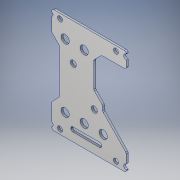
# Autodesk Inventor part: End Plate - 18S
Saved by Autodesk Inventor 2017 (Build 210142000, 142)
## iProperties
Created: 2021-03-03
Part Number: End Plate - 18S
Material: Aluminum 6061
Document SubType Name: Modeling
Designer: Win240
Density: 2.7 g/cm^3
Appearance: Aluminum - Flat
Mass: 164.512 g
Surface Area: 306.178 cm^2
Volume: 60.9303 cm^3
Author: Win240
Autodesk Inventor part; units mm, degrees
ref_plane "YZ Plane" through (0, 0, 0) normal (1, 0, 0) x (0, 1, 0)
ref_plane "XZ Plane" through (0, 0, 0) normal (0, 1, 0) x (-1, 0, 0)
ref_plane "XY Plane" through (0, 0, 0) normal (0, 0, 1) x (1, 0, 0)
sketch "Sketch1" plane through (0, 0, 0) normal (0, 0, 1) x (1, 0, 0)
  line L0 (0, 0) -> (119, 0)
  line L1 (119, 0) -> (119, -24.5)
  line L2 (119, -165) -> (0, -165)
  line L3 (0, -165) -> (0, 0)
  arc A0 (0, -11.373) -> (0, -3.627) centre (-1, -7.5) ccw
  arc A1 (119, -3.627) -> (119, -11.373) centre (120, -7.5) ccw
  arc A2 (119, -153.627) -> (119, -161.373) centre (120, -157.5) ccw
  arc A3 (0, -161.373) -> (0, -153.627) centre (-1, -157.5) ccw
  line L4 (-1, -7.5) -> (120, -7.5) construction
  line L5 (120, -7.5) -> (120, -157.5) construction
  line L6 (120, -157.5) -> (-1, -157.5) construction
  line L7 (-1, -157.5) -> (-1, -7.5) construction
  line L8 (-1, -7.5) -> (0, -3.627) construction
  line L9 (120, -7.5) -> (119, -3.627) construction
  line L10 (59.5, -7.5) -> (59.5, 0) construction
  line L11 (59.5, -157.5) -> (59.5, -165) construction
  circle A4 centre (22, -31) radius 6.5
  circle A5 centre (52, -31) radius 6.5
  arc A6 (82, -24.5) -> (78.25, -36.3092) centre (82, -31) ccw
  circle A7 centre (82, -131) radius 6.5
  circle A8 centre (52, -131) radius 6.5
  circle A9 centre (22, -131) radius 6.5
  line L12 (22, -31) -> (52, -31) construction
  line L13 (52, -31) -> (82, -31) construction
  line L14 (82, -31) -> (82, -131) construction
  line L15 (82, -131) -> (52, -131) construction
  line L16 (52, -131) -> (22, -131) construction
  line L17 (22, -131) -> (22, -31) construction
  circle A10 centre (68, -104) radius 4.75
  circle A11 centre (35, -58) radius 4.75
  circle A12 centre (102, -7.5) radius 4
  line L18 (67, -44.5) -> (73, -44.5)
  line L19 (73, -44.5) -> (73, -70.5)
  line L20 (73, -70.5) -> (67, -70.5)
  line L21 (67, -70.5) -> (67, -44.5)
  line L22 (82, -24.5) -> (119, -24.5)
  line L23 (81, -41.6184) -> (81, -92.5)
  arc A13 (81, -53.25) -> (81, -62.75) centre (81, -58) ccw construction
  circle A14 centre (48, -104) radius 4.75 construction
  line L24 (48, -104) -> (68, -104) construction
  line L25 (35, -58) -> (81, -58) construction
  arc A15 (81, -41.6184) -> (78.25, -36.3092) centre (74.5, -41.6184) ccw
  line L26 (81, -92.5) -> (91, -92.5)
  line L27 (91, -92.5) -> (91, -110.5)
  line L28 (91, -110.5) -> (119, -110.5)
  arc A16 (82, -37.5) -> (82, -24.5) centre (82, -31) ccw construction
  arc A17 (78.25, -36.3092) -> (82, -37.5) centre (82, -31) ccw construction
  arc A18 (82, -53.3565) -> (81, -53.25) centre (81, -58) ccw construction
  arc A19 (82, -62.6435) -> (82, -53.3565) centre (81, -58) ccw construction
  arc A20 (81, -62.75) -> (82, -62.6435) centre (81, -58) ccw construction
  line L29 (119, -24.5) -> (119, -110.5) construction
  line L30 (119, -110.5) -> (119, -165)
  circle A21 centre (102, -157.5) radius 4
  line L31 (102, -7.5) -> (102, -157.5) construction
  circle A22 centre (14, -7.5) radius 4
  line L32 (102, -7.5) -> (119, -3.627) construction
  line L33 (14, -7.5) -> (0, -3.627) construction
  circle A23 centre (14, -157.5) radius 4
  line L34 (14, -157.5) -> (14, -7.5) construction
  dimension "d0" = 119
  dimension "d1" = 165
  dimension "d2" = 150
  dimension "d3" = 121
  dimension "d4" = 4
  dimension "d5" = 13
  dimension "d6" = 30
  dimension "d7" = 100
  dimension "d9" = 23
  dimension "d10" = 9.5
  dimension "d11" = 36
  dimension "d12" = 69
  dimension "d15" = 103
  dimension "d16" = 63
  dimension "d17" = 37
  dimension "d18" = 68
  dimension "d19" = 74
  dimension "d20" = 82
  dimension "d21" = 82
  dimension "d22" = 49
  dimension "d23" = 85
  dimension "d24" = 92
  dimension "d25" = 103
  dimension "d44" = 26.5
  dimension "d45" = 99.5
  dimension "d46" = 53.5
  dimension "d54" = 88
  constraints: 70 end point, 24 centre point, 24 point on circle, 22 point on line, 16 equal radius, 13 horizontal, 9 vertical, 6 parallel, 4 midpoint, 4 perpendicular, 4 tangent, 3 equal length
  measures "d0" distance of L2.start L2.end
  measures "d1" distance of L0.end L2.start
  measures "d2" distance of L4.end L5.end
  measures "d3" distance of L5.end L6.end
  measures "d4" radius of A0
  measures "d5" diameter of A4
  measures "d6" distance of L12.start L12.end
  measures "d7" distance of L16.end L12.start
  measures "d9" distance between parallel lines of L17 L7
  measures "d10" diameter of A11
  measures "d11" distance from line of L25.start L7
  measures "d12" distance from line of L24.end L7
  measures "d15" distance of L31.start L4.start
  measures "d16" distance between parallel lines of L20 L4
  measures "d17" distance between parallel lines of L18 L4
  measures "d18" distance between parallel lines of L21 L7
  measures "d19" distance between parallel lines of L19 L7
  measures "d20" distance between parallel lines of L7 L23
  measures "d21" distance from line of L7 L25.end
  measures "d22" distance from line of L24.start L7
  measures "d23" distance between parallel lines of L4 L26
  measures "d24" distance between parallel lines of L7 L27
  measures "d25" distance between parallel lines of L4 L28
  measures "d44" distance between parallel lines of L16 L6
  measures "d45" distance between parallel lines of L25 L6
  measures "d46" distance between parallel lines of L6 L24
  measures "d54" distance between parallel lines of L31 L34
extrude "Mechanical Holes" add sketch "Sketch1" along normal blind 3.175 contours L0 L1 A1 L22 A6 A15 L23 L26 L27 L28 L30 A2 L2 L3 A3 A0
sketch "Sketch2" plane through (0, 0, 3.175) normal (0, 0, 1) x (1, 0, 0)
  line L0 (0, -11.373) -> (0, -153.627) projected
  line L1 (119, 0) -> (0, 0) projected
  line L2 (0, -165) -> (119, -165) projected
  line L3 (79.3158, -151.5) -> (31.0925, -151.5)
  line L4 (31.0925, -151.5) -> (31.0925, -144.5)
  line L5 (31.0925, -144.5) -> (79.3158, -144.5)
  line L6 (79.3158, -144.5) -> (79.3158, -151.5)
  line L7 (3, -44.5) -> (13, -44.5)
  line L8 (13, -44.5) -> (13, -72.5)
  line L9 (13, -72.5) -> (3, -72.5)
  line L10 (3, -72.5) -> (3, -44.5)
  arc A0 (0, -11.373) -> (0, -3.627) centre (-1, -7.5) ccw construction
  line L11 (13, -86.5) -> (3, -86.5)
  line L12 (3, -86.5) -> (3, -114.5)
  line L13 (3, -114.5) -> (13, -114.5)
  line L14 (13, -114.5) -> (13, -86.5)
  arc A1 (0, -161.373) -> (0, -153.627) centre (-1, -157.5) ccw construction
  circle A2 centre (14, -157.5) radius 4 construction
  circle A3 centre (52, -131) radius 6.5 construction
  line L15 (47.1703, -126.6498) -> (16.9721, -160.177) construction
  circle A4 centre (102, -157.5) radius 4 construction
  line L16 (99.5036, -160.6253) -> (56.0567, -125.9213) construction
  dimension "d28" = 4
  dimension "d29" = 10
  dimension "d30" = 65
  dimension "d31" = 79
  dimension "d32" = 28
  dimension "d47" = 6
  dimension "d48" = 13
  constraints: 28 end point, 6 parallel, 3 collinear, 3 horizontal, 3 perpendicular, 2 point on circle, 2 point on line, 2 tangent, 6 other
  measures "d28" distance from line of L10 A0.centre
  measures "d29" distance of L7.start L7.end
  measures "d30" distance from line of L9 A0.centre
  measures "d31" distance from line of L11 A0.centre
  measures "d32" distance of L7.end L8.end
  measures "d47" distance from line of A1.centre L3
  measures "d48" distance from line of A1.centre L5
extrude "Air Holes" cut sketch "Sketch2" against normal up to surface (3.175 mm away)
sketch "Sketch4" plane through (0, 0, 0) normal (0, 0, -1) x (-1, 0, 0)
  line L0 (-119, -153.627) -> (-119, -110.5) projected
  arc A0 (-119, -161.373) -> (-119, -153.627) centre (-120, -157.5) ccw projected
  line L1 (-119, -165) -> (-119, -161.373) projected
  line L2 (-118, -138.2788) -> (-118, -154.0359)
  line L3 (-118, -160.9641) -> (-118, -165)
  line L4 (-118, -165) -> (-119, -165)
  line L5 (-119, -110.5) -> (-91, -110.5) projected
  line L6 (-118, -138.2788) -> (-91, -110.5)
  circle A1 centre (-68, -104) radius 4.75 projected
  line L7 (-68, -104) -> (-120, -157.5) construction
  line L8 (-91, -110.5) -> (-81, -100.2115)
  line L9 (-91, -110.5) -> (-91, -92.5) projected
  line L10 (-91, -92.5) -> (-81, -92.5) projected
  line L11 (-81, -92.5) -> (-81, -100.2115)
  point P0 (0, 0)
  dimension "d41" = 1
  constraints: 14 end point, 3 vertical, 2 collinear, 2 point on circle, 1 horizontal, 1 parallel
  measures "d41" distance of L3.end L1.start
extrude "Increase Airflow Below Connector" cut sketch "Sketch4" against normal up to surface (3.175 mm away) contours L9 L10 L11 L8 | L0 L5 L6 L2 A0 | A0 L3 L4 L1
sketch "Sketch5" plane through (0, 0, 0) normal (0, 0, -1) x (-1, 0, 0)
  line L0 (-81, -100.2115) -> (-118, -138.2788) construction
  line L1 (-67, -44.5) -> (-67, -70.5) projected
  line L2 (-67, -77.8932) -> (-81, -92.2971)
  line L3 (-81, -41.6184) -> (-81, -100.2115) projected
  arc A0 (-78.25, -36.3092) -> (-82, -24.5) centre (-82, -31) ccw projected
  arc A1 (-78.25, -36.3092) -> (-81, -41.6184) centre (-74.5, -41.6184) ccw projected
  line L4 (-67, -37.1068) -> (-77.3389, -26.4696)
  line L5 (-13, -114.5) -> (-13, -86.5) projected
  line L6 (-13, -72.5) -> (-13, -44.5) projected
  line L7 (0, -11.373) -> (0, -153.627) projected
  line L8 (-13, -114.5) -> (0, -127.875)
  line L9 (-13, -86.5) -> (-13, -72.5)
  line L10 (-13, -44.5) -> (0, -31.125)
  line L11 (-67, -44.5) -> (-67, -37.1068)
  line L12 (-67, -70.5) -> (-67, -77.8932)
  point P0 (0, 0)
  constraints: 14 end point, 3 parallel, 3 point on line, 2 equal length, 2 vertical, 1 point on circle, 1 tangent
extrude "Extrusion4" cut sketch "Sketch5" against normal up to surface (3.175 mm away)
sketch "Sketch6" plane through (0, 0, 3.175) normal (0, 0, 1) x (1, 0, 0)
  line L0 (0, -165) -> (118, -165) projected
  line L1 (118, -165) -> (118, 0)
  line L2 (119, 0) -> (0, 0) projected
  line L3 (1, 0) -> (1, -165)
  line L4 (0, 0) -> (0, -165)
  line L5 (119, 0) -> (119, -165)
  line L6 (118, -165) -> (119, -165)
  dimension "d51" = 1
  constraints: 10 end point, 3 point on line, 3 vertical, 1 horizontal
  measures "d51" distance from line of L0.start L3
extrude "Extrusion5" cut sketch "Sketch6" against normal up to surface (3.175 mm away) contours L4 L2 L3 L0 | L1 L2 L5 L6
fillet "Fillet1" radius 3 18 edges at (13, -114.5, 1.5875) (31.0925, -151.5, 1.5875) (79.3158, -151.5, 1.5875) (13, -44.5, 1.5875) (79.3158, -144.5, 1.5875) (31.0925, -144.5, 1.5875) (118, -165, 1.5875) (118, -138.2788, 1.5875) (81, -100.2115, 1.5875) (81, -92.2971, 1.5875) (67, -77.8932, 1.5875) (67, -37.1068, 1.5875) (1, -126.8462, 1.5875) (1, -165, 1.5875) (1, -32.1538, 1.5875) (1, 0, 1.5875) (118, 0, 1.5875) (118, -24.5, 1.5875)
sketch "Sketch7" plane through (0, 0, 3.175) normal (0, 0, 1) x (1, 0, 0)
  arc A0 (118, -4.0359) -> (118, -10.9641) centre (120, -7.5) ccw projected
  arc A1 (118, -3.5) -> (118, -11.5) centre (118, -7.5) ccw
  line L0 (118, -7.5) -> (120, -7.5) construction
  line L1 (118, -4.0359) -> (118, -3) projected
  line L2 (118, -21.5) -> (118, -10.9641) projected
  line L3 (118, -162) -> (118, -160.9641) projected
  line L4 (118, -154.0359) -> (118, -139.4966) projected
  arc A2 (118, -154.0359) -> (118, -160.9641) centre (120, -157.5) ccw projected
  arc A3 (118, -153.5) -> (118, -161.5) centre (118, -157.5) ccw
  line L5 (118, -157.5) -> (120, -157.5) construction
  point P0 (0, 0)
  constraints: 4 end point, 4 point on circle, 4 point on line, 2 centre point, 2 equal radius, 2 horizontal, 2 line through centre
extrude "Extrusion6" cut sketch "Sketch7" against normal up to surface (3.175 mm away)
body "Solid1"
